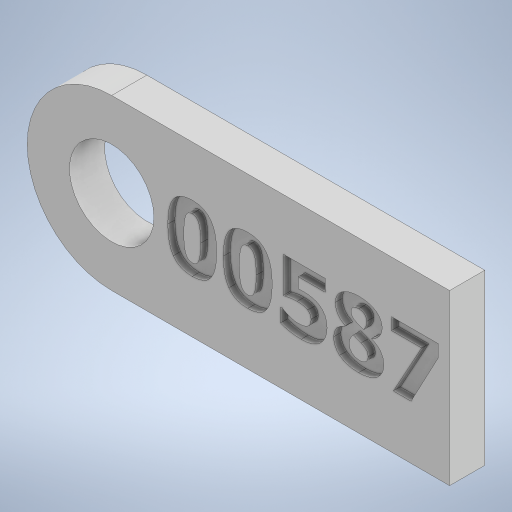
# Autodesk Inventor part: T3H Asset Tag
Saved by Autodesk Inventor 2024 (Build 280153000, 153)
## iProperties
Created: 2024-12-23
Part Number: T3H Asset Tag
Material: Generic
Document SubType Name: Modeling
Designer: dwise
Density: 1 g/cm^3
Appearance: Default
Author: dwise
Autodesk Inventor part; units mm, degrees
ref_plane "YZ Plane" through (0, 0, 0) normal (1, 0, 0) x (0, 1, 0)
ref_plane "XZ Plane" through (0, 0, 0) normal (0, 1, 0) x (-1, 0, 0)
ref_plane "XY Plane" through (0, 0, 0) normal (0, 0, 1) x (1, 0, 0)
sketch "Sketch1" plane through (0, 0, 0) normal (0, 0, 1) x (1, 0, 0)
  line L0 (0, 0) -> (76.2, 0)
  line L1 (76.2, 0) -> (76.2, -30.48)
  line L2 (76.2, -30.48) -> (0, -30.48)
  line L3 (0, -30.48) -> (0, 0)
  dimension "d0" = 76.2
  dimension "d1" = 30.48
  constraints: 8 end point, 2 parallel, 1 horizontal, 1 perpendicular
  measures "d0" distance of L1.end L2.end
  measures "d1" distance of L0.end L1.end
extrude "Extrusion1" add sketch "Sketch1" along normal blind 6.35
fillet "Fillet1" radius 15.24 2 edges at (0, 0, 3.175) (0, -30.48, 3.175)
sketch "Sketch5" plane through (0, 0, 6.35) normal (0, 0, 1) x (1, 0, 0)
  arc A0 (15.24, 0) -> (15.24, -30.48) centre (15.24, -15.24) ccw projected
  circle A1 centre (15.24, -15.24) radius 7.62
  point P0 (0, 0)
  dimension "d11" = 15.24
  constraints: 1 centre point, 1 coincident
  measures "d11" diameter of A1
extrude "Extrusion4" cut sketch "Sketch5" against normal blind 6.35
sketch "Sketch4" plane through (0, 0, 6.35) normal (0, 0, 1) x (1, 0, 0)
  line L0 (24.7701, -9.0598) -> (87.4746, -9.0598) construction
  line L1 (87.4746, -9.0598) -> (87.4746, -34.6158) construction
  line L2 (87.4746, -34.6158) -> (24.7701, -34.6158) construction
  line L3 (24.7701, -34.6158) -> (24.7701, -9.0598) construction
  spline S0 degree 2 poles (34.1808, -15.0341) (34.1808, -16.5161) (33.7084, -18.7391) (33.1805, -19.4894) knots 0 0 0 1 2 2 2
  spline S1 degree 2 poles (33.1805, -19.4894) (32.6618, -20.2304) (30.9853, -20.9899) (29.7811, -20.9899) knots 0 0 0 1 2 2 2
  spline S2 degree 2 poles (29.7811, -20.9899) (28.5677, -20.9899) (26.9005, -20.2304) (26.3725, -19.4709) knots 0 0 0 1 2 2 2
  spline S3 degree 2 poles (26.3725, -19.4709) (25.8445, -18.7206) (25.3721, -16.5161) (25.3721, -15.0341) knots 0 0 0 1 2 2 2
  spline S4 degree 2 poles (25.3721, -15.0341) (25.3721, -13.515) (25.8445, -11.3661) (26.3818, -10.5881) knots 0 0 0 1 2 2 2
  spline S5 degree 2 poles (26.3818, -10.5881) (26.919, -9.8285) (28.614, -9.0875) (29.7811, -9.0875) knots 0 0 0 1 2 2 2
  spline S6 degree 2 poles (29.7811, -9.0875) (31.013, -9.0875) (32.6618, -9.8656) (33.1897, -10.6344) knots 0 0 0 1 2 2 2
  spline S7 degree 2 poles (33.1897, -10.6344) (33.7084, -11.3847) (34.1808, -13.5984) (34.1808, -15.0341) knots 0 0 0 1 2 2 2
  spline S8 degree 2 poles (31.3002, -15.0341) (31.3002, -12.913) (30.6055, -11.1994) (29.7811, -11.1994) knots 0 0 0 1 2 2 2
  spline S9 degree 2 poles (29.7811, -11.1994) (28.9568, -11.1994) (28.2528, -12.913) (28.2528, -15.0434) knots 0 0 0 1 2 2 2
  spline S10 degree 2 poles (28.2528, -15.0434) (28.2528, -17.1367) (28.9568, -18.8781) (29.7811, -18.8781) knots 0 0 0 1 2 2 2
  spline S11 degree 2 poles (29.7811, -18.8781) (30.5962, -18.8781) (31.3002, -17.1367) (31.3002, -15.0341) knots 0 0 0 1 2 2 2
  spline S12 degree 2 poles (44.1937, -15.0341) (44.1937, -16.5161) (43.7213, -18.7391) (43.1933, -19.4894) knots 0 0 0 1 2 2 2
  spline S13 degree 2 poles (43.1933, -19.4894) (42.6746, -20.2304) (40.9981, -20.9899) (39.794, -20.9899) knots 0 0 0 1 2 2 2
  spline S14 degree 2 poles (39.794, -20.9899) (38.5806, -20.9899) (36.9133, -20.2304) (36.3853, -19.4709) knots 0 0 0 1 2 2 2
  spline S15 degree 2 poles (36.3853, -19.4709) (35.8574, -18.7206) (35.385, -16.5161) (35.385, -15.0341) knots 0 0 0 1 2 2 2
  spline S16 degree 2 poles (35.385, -15.0341) (35.385, -13.515) (35.8574, -11.3661) (36.3946, -10.5881) knots 0 0 0 1 2 2 2
  spline S17 degree 2 poles (36.3946, -10.5881) (36.9318, -9.8285) (38.6269, -9.0875) (39.794, -9.0875) knots 0 0 0 1 2 2 2
  spline S18 degree 2 poles (39.794, -9.0875) (41.0259, -9.0875) (42.6746, -9.8656) (43.2026, -10.6344) knots 0 0 0 1 2 2 2
  spline S19 degree 2 poles (43.2026, -10.6344) (43.7213, -11.3847) (44.1937, -13.5984) (44.1937, -15.0341) knots 0 0 0 1 2 2 2
  spline S20 degree 2 poles (41.313, -15.0341) (41.313, -12.913) (40.6183, -11.1994) (39.794, -11.1994) knots 0 0 0 1 2 2 2
  spline S21 degree 2 poles (39.794, -11.1994) (38.9696, -11.1994) (38.2656, -12.913) (38.2656, -15.0434) knots 0 0 0 1 2 2 2
  spline S22 degree 2 poles (38.2656, -15.0434) (38.2656, -17.1367) (38.9696, -18.8781) (39.794, -18.8781) knots 0 0 0 1 2 2 2
  spline S23 degree 2 poles (39.794, -18.8781) (40.6091, -18.8781) (41.313, -17.1367) (41.313, -15.0341) knots 0 0 0 1 2 2 2
  spline S24 degree 2 poles (54.0953, -16.8774) (54.0953, -17.7758) (53.484, -19.2949) (52.8819, -19.8414) knots 0 0 0 1 2 2 2
  spline S25 degree 2 poles (52.8819, -19.8414) (52.2799, -20.3879) (50.6311, -20.9899) (49.427, -20.9899) knots 0 0 0 1 2 2 2
  spline S26 degree 2 poles (49.427, -20.9899) (48.1488, -20.9807) (46.3148, -20.5639) (45.7127, -20.2952) knots 0 0 0 1 2 2 2
  line L4 (45.7127, -20.2952) -> (45.7127, -17.8036)
  line L5 (45.7127, -17.8036) -> (45.9721, -17.8036)
  spline S27 degree 2 poles (45.9721, -17.8036) (46.1944, -17.924) (46.7316, -18.2389) (47.1669, -18.4057) knots 0 0 0 1 2 2 2
  spline S28 degree 2 poles (47.1669, -18.4057) (47.5745, -18.5631) (48.4174, -18.7762) (48.9268, -18.7762) knots 0 0 0 1 2 2 2
  spline S29 degree 2 poles (48.9268, -18.7762) (49.3714, -18.7762) (50.4088, -18.5539) (50.7238, -18.2575) knots 0 0 0 1 2 2 2
  spline S30 degree 2 poles (50.7238, -18.2575) (50.9553, -18.0259) (51.2147, -17.4609) (51.2147, -16.9885) knots 0 0 0 1 2 2 2
  spline S31 degree 2 poles (51.2147, -16.9885) (51.2147, -16.581) (50.8812, -16.0067) (50.6126, -15.8307) knots 0 0 0 1 2 2 2
  spline S32 degree 2 poles (50.6126, -15.8307) (50.2236, -15.5713) (49.1121, -15.4231) (48.7138, -15.4231) knots 0 0 0 1 2 2 2
  spline S33 degree 2 poles (48.7138, -15.4231) (48.0839, -15.4231) (46.8891, -15.6269) (46.4537, -15.7381) knots 0 0 0 1 2 2 2
  line L6 (46.4537, -15.7381) -> (46.2036, -15.7381)
  line L7 (46.2036, -15.7381) -> (46.2036, -9.3191)
  line L8 (46.2036, -9.3191) -> (53.7804, -9.3191)
  line L9 (53.7804, -9.3191) -> (53.7804, -11.4773)
  line L10 (53.7804, -11.4773) -> (48.9176, -11.4773)
  line L11 (48.9176, -11.4773) -> (48.9176, -13.3761)
  spline S34 degree 2 poles (48.9176, -13.3761) (49.1491, -13.3576) (49.7883, -13.3391) (49.9642, -13.3391) knots 0 0 0 1 2 2 2
  spline S35 degree 2 poles (49.9642, -13.3391) (50.7886, -13.3391) (52.178, -13.6725) (52.7245, -14.0152) knots 0 0 0 1 2 2 2
  spline S36 degree 2 poles (52.7245, -14.0152) (53.3729, -14.4413) (54.0953, -15.8585) (54.0953, -16.8774) knots 0 0 0 1 2 2 2
  spline S37 degree 2 poles (64.3397, -17.572) (64.3397, -18.3038) (63.7284, -19.5728) (63.1449, -20.0359) knots 0 0 0 1 2 2 2
  spline S38 degree 2 poles (63.1449, -20.0359) (62.5613, -20.499) (60.8848, -21.0177) (59.8011, -21.0177) knots 0 0 0 1 2 2 2
  spline S39 degree 2 poles (59.8011, -21.0177) (58.6433, -21.0177) (56.9112, -20.4898) (56.3554, -20.0359) knots 0 0 0 1 2 2 2
  spline S40 degree 2 poles (56.3554, -20.0359) (55.8089, -19.582) (55.2902, -18.3501) (55.2902, -17.6647) knots 0 0 0 1 2 2 2
  spline S41 degree 2 poles (55.2902, -17.6647) (55.2902, -16.6828) (56.3739, -15.3768) (57.4021, -14.9415) knots 0 0 0 1 2 2 2
  line L12 (57.4021, -14.9415) -> (57.4021, -14.8952)
  spline S42 degree 2 poles (57.4021, -14.8952) (56.3925, -14.4042) (55.5959, -13.0056) (55.5959, -12.1442) knots 0 0 0 1 2 2 2
  spline S43 degree 2 poles (55.5959, -12.1442) (55.5959, -11.5143) (56.1516, -10.4121) (56.6981, -9.9767) knots 0 0 0 1 2 2 2
  spline S44 degree 2 poles (56.6981, -9.9767) (57.2261, -9.5599) (58.8285, -9.0598) (59.8289, -9.0598) knots 0 0 0 1 2 2 2
  spline S45 degree 2 poles (59.8289, -9.0598) (60.8848, -9.0598) (62.4594, -9.5136) (62.9689, -9.8841) knots 0 0 0 1 2 2 2
  spline S46 degree 2 poles (62.9689, -9.8841) (63.4876, -10.2546) (64.0433, -11.3291) (64.0433, -11.9497) knots 0 0 0 1 2 2 2
  spline S47 degree 2 poles (64.0433, -11.9497) (64.0433, -12.7648) (63.0986, -14.0708) (62.126, -14.5247) knots 0 0 0 1 2 2 2
  line L13 (62.126, -14.5247) -> (62.126, -14.5617)
  spline S48 degree 2 poles (62.126, -14.5617) (63.2653, -15.0248) (64.3397, -16.5254) (64.3397, -17.572) knots 0 0 0 1 2 2 2
  spline S49 degree 2 poles (61.5054, -17.6925) (61.5054, -17.1274) (61.0237, -16.5346) (60.2457, -16.1549) knots 0 0 0 1 2 2 2
  spline S50 degree 2 poles (60.2457, -16.1549) (60.0234, -16.053) (59.1805, -15.7288) (58.8563, -15.5899) knots 0 0 0 1 2 2 2
  spline S51 degree 2 poles (58.8563, -15.5899) (58.5599, -15.8863) (58.0875, -16.7755) (58.0875, -17.3034) knots 0 0 0 1 2 2 2
  spline S52 degree 2 poles (58.0875, -17.3034) (58.0875, -18.1) (59.1064, -19.0541) (59.9308, -19.0541) knots 0 0 0 1 2 2 2
  spline S53 degree 2 poles (59.9308, -19.0541) (60.1623, -19.0541) (60.7366, -18.9059) (60.9589, -18.7577) knots 0 0 0 1 2 2 2
  spline S54 degree 2 poles (60.9589, -18.7577) (61.209, -18.5817) (61.5054, -18.1) (61.5054, -17.6925) knots 0 0 0 1 2 2 2
  spline S55 degree 2 poles (61.2553, -12.2831) (61.2553, -11.6996) (60.4865, -11.0049) (59.8289, -11.0049) knots 0 0 0 1 2 2 2
  spline S56 degree 2 poles (59.8289, -11.0049) (59.199, -11.0049) (58.4302, -11.6347) (58.4302, -12.0979) knots 0 0 0 1 2 2 2
  spline S57 degree 2 poles (58.4302, -12.0979) (58.4302, -12.5517) (58.8934, -13.1168) (59.3843, -13.3483) knots 0 0 0 1 2 2 2
  spline S58 degree 2 poles (59.3843, -13.3483) (59.5973, -13.4595) (60.1901, -13.691) (60.681, -13.8763) knots 0 0 0 1 2 2 2
  spline S59 degree 2 poles (60.681, -13.8763) (60.9774, -13.4873) (61.2553, -12.7555) (61.2553, -12.2831) knots 0 0 0 1 2 2 2
  line L14 (74.1303, -11.5884) -> (69.2489, -20.7491)
  line L15 (69.2489, -20.7491) -> (66.0626, -20.7491)
  line L16 (66.0626, -20.7491) -> (71.1662, -11.4773)
  line L17 (71.1662, -11.4773) -> (65.7199, -11.4773)
  line L18 (65.7199, -11.4773) -> (65.7199, -9.3191)
  line L19 (65.7199, -9.3191) -> (74.1303, -9.3191)
  line L20 (74.1303, -9.3191) -> (74.1303, -11.5884)
  point P0 (0, 0)
  constraints: 2 other
extrude "Extrusion3" cut sketch "Sketch4" against normal blind 1.27
body "Solid1"
